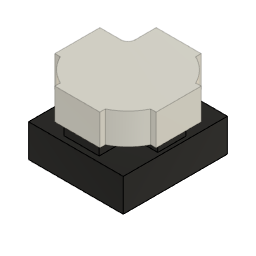
Marquardt_6425_0101 (Autodesk Fusion 360 design; units mm, degrees)
Autodesk Fusion 360 part; units mm, degrees
sketch "Sketch1" plane through (0, 0, 0) normal (0, 0, 1) x (1, 0, 0) in component "Base"
  line L0 (6.725, -7.4) -> (-6.725, -7.4)
  line L1 (-6.725, -7.4) -> (-6.725, 7.4)
  line L2 (-6.725, 7.4) -> (6.725, 7.4)
  line L3 (6.725, 7.4) -> (6.725, -7.4)
  line L4 (6.725, -7.4) -> (-6.725, 7.4) construction
  line L5 (-6.725, -7.4) -> (6.725, 7.4) construction
  dimension "d1" = 13.45
  dimension "d2" = 14.8
  constraint horizontal L0
  constraint perpendicular L0 L1
  constraint parallel L0 L2
  constraint parallel L1 L3
  constraint coincident L4 origin
  constraint coincident L5 origin
  measures "d1" distance of L1.end L2.end
  measures "d2" distance of L0.end L1.end
extrude "Extrude1" add sketch "Sketch1" along normal blind 4.65 makes body 1 in component "Base"
sketch "Sketch2" plane through (0, 0, 4.65) normal (0, 0, 1) x (-1, 0, 0) in component "Base"
  line L0 (-6.725, -7.4) -> (6.725, -7.4)
  line L1 (6.725, -7.4) -> (6.725, 7.4)
  line L2 (6.725, 7.4) -> (-6.725, 7.4)
  line L3 (-6.725, 7.4) -> (-6.725, -7.4)
  line L4 (0, -7.4) -> (0, 7.4) construction
  line L5 (6.725, 0) -> (-6.725, 0) construction
  line L6 (2.5, -6.6) -> (1.8392, -6.6)
  line L7 (1.8392, -6.6) -> (-2.5, -6.6)
  line L8 (-2.5, -6.6) -> (-2.5, -2)
  line L9 (-2.5, -2) -> (-6.225, -2)
  line L10 (-6.225, -2) -> (-6.225, 2)
  line L11 (-6.225, 2) -> (-2.5, 2)
  line L12 (-2.5, 2) -> (-2.5, 6.6)
  line L13 (-2.5, 6.6) -> (2.5, 6.6)
  line L14 (2.5, 6.6) -> (2.5, 2)
  line L15 (2.5, 2) -> (6.225, 2)
  line L16 (6.225, 2) -> (6.225, -2)
  line L17 (6.225, -2) -> (2.5, -2)
  line L18 (2.5, -2) -> (2.5, -6.6)
  dimension "d5" = 4
  dimension "d6" = 5
  dimension "d7" = 0.8
  dimension "d8" = 0.8
  dimension "d9" = 0.5
  constraint midpoint L0 L4.start
  constraint midpoint L2 L4.end
  constraint midpoint L1 L5.start
  constraint midpoint L3 L5.end
  constraint horizontal L6
  constraint perpendicular L4 L7
  constraint perpendicular L7 L8
  constraint perpendicular L8 L9
  constraint perpendicular L7 L10
  constraint perpendicular L10 L11
  constraint perpendicular L11 L12
  constraint perpendicular L10 L13
  constraint perpendicular L11 L14
  constraint perpendicular L14 L15
  constraint perpendicular L5 L16
  constraint perpendicular L16 L17
  constraint perpendicular L5 L18
  constraint equal L12 L14
  constraint equal L8 L18
  constraint equal L15 L17
  constraint equal L9 L15
  constraint equal L9 L11
  constraint symmetric L5 L9.end L10.end
  constraint symmetric L4 L12.end L13.end
  measures "d5" distance of L9.end L10.end
  measures "d6" distance of L12.end L13.end
  measures "d7" vertical distance of L2.end L12.end
  measures "d8" vertical distance of L0.start L7.end
  measures "d9" horizontal distance of L1.end L15.end
extrude "Extrude2" add sketch "Sketch2" along normal blind 4 contours L6 L7 L8 L9 L10 L11 L12 L13 L14 L15 L16 L17 L18 bodies 1 in component "Base"
sketch "Sketch3" plane through (0, 0, 0) normal (0, 0, -1) x (1, 0, 0) in component "Base"
  line L0 (-6.725, -7.4) -> (6.725, -7.4)
  line L1 (6.725, -7.4) -> (6.725, 7.4)
  line L2 (6.725, 7.4) -> (-6.725, 7.4)
  line L3 (-6.725, 7.4) -> (-6.725, -7.4)
  circle A0 centre (5.08, -5.08) radius 0.4
  circle A1 centre (-5.08, 5.08) radius 0.4
  dimension "d12" = 0.8
  dimension "d13" = 5.08
  dimension "d14" = 5.08
  dimension "d15" = 5.08
  dimension "d16" = 5.08
  constraint equal A0 A1
  measures "d12" diameter of A0
  measures "d13" horizontal distance of origin A0.centre
  measures "d14" vertical distance of origin A0.centre
  measures "d15" horizontal distance of origin A1.centre
  measures "d16" vertical distance of origin A1.centre
extrude "Extrude3" add sketch "Sketch3" along normal blind 1.5 contours A0 | A1 bodies 1 in component "Base"
chamfer "Chamfer1" distance 0.25 angle 45 2 edges at (-5.4529, -4.9354, -1.5) (4.7071, 5.2246, -1.5) on bodies 1 in component "Base"
sketch "Sketch4" plane through (0, 0, 4.65) normal (0, 0, 1) x (-1, 0, 0) in component "Base"
  line L0 (2.5, -2) -> (2.5, -6.6)
  line L1 (2.5, -6.6) -> (-2.5, -6.6)
  line L2 (-2.5, -6.6) -> (-2.5, -2)
  line L3 (-2.5, -2) -> (-6.225, -2)
  line L4 (-6.225, -2) -> (-6.225, 2)
  line L5 (-6.225, 2) -> (-2.5, 2)
  line L6 (-2.5, 2) -> (-2.5, 6.6)
  line L7 (-2.5, 6.6) -> (2.5, 6.6)
  line L8 (2.5, 6.6) -> (2.5, 2)
  line L9 (2.5, 2) -> (6.225, 2)
  line L10 (6.225, 2) -> (6.225, -2)
  line L11 (6.225, -2) -> (2.5, -2)
  line L12 (-6.725, -7.4) -> (6.725, -7.4)
  line L13 (6.725, -7.4) -> (6.725, 7.4)
  line L14 (6.725, 7.4) -> (-6.725, 7.4)
  line L15 (-6.725, 7.4) -> (-6.725, -7.4)
  circle A0 centre (4.15, -5.95) radius 0.5
  circle A1 centre (5.95, -4.15) radius 0.5
  dimension "d20" = 1
  dimension "d21" = 4.15
  dimension "d22" = 5.95
  dimension "d23" = 4.15
  dimension "d24" = 5.95
  constraint equal A0 A1
  measures "d20" diameter of A0
  measures "d21" horizontal distance of origin A0.centre
  measures "d22" horizontal distance of origin A1.centre
  measures "d23" vertical distance of origin A1.centre
  measures "d24" vertical distance of origin A0.centre
extrude "Extrude4" cut sketch "Sketch4" against normal through all contours A0 | A1 bodies 1 in component "Base"
ref_plane "WorkPlane1" through (0, 0, 10.7) normal (0, 0, -1) x (-1, 0, 0) in component "Plunger"
sketch "Sketch1 (2)" plane through (0, 0, 10.7) normal (0, 0, -1) x (1, 0, 0) in component "Plunger"
  line L0 (7.2, 7.2) -> (-7.2, 7.2) construction
  line L1 (-7.2, 7.2) -> (-7.2, -7.2) construction
  line L2 (-7.2, -7.2) -> (7.2, -7.2) construction
  line L3 (7.2, -7.2) -> (7.2, 7.2) construction
  line L4 (7.2, 7.2) -> (-7.2, -7.2) construction
  line L5 (-7.2, 7.2) -> (7.2, -7.2) construction
  line L6 (0, -7.2) -> (0, 7.2) construction
  line L7 (-7.2, 0) -> (7.2, 0) construction
  line L8 (-3.2, 7.2) -> (3.2, 7.2)
  line L9 (-3.2, -7.2) -> (3.2, -7.2)
  line L10 (7.2, -3.2) -> (7.2, 3.2)
  line L11 (-7.2, 3.2) -> (-7.2, -3.2)
  arc A0 (6.4219, 3.2) -> (3.2, 6.4219) centre (0, 0) ccw
  line L12 (7.2, 3.2) -> (6.4219, 3.2)
  line L13 (3.2, 7.2) -> (3.2, 6.4219)
  arc A1 (3.2, -6.4219) -> (6.4219, -3.2) centre (0, 0) ccw
  arc A2 (-3.2, 6.4219) -> (-6.4219, 3.2) centre (0, 0) ccw
  line L14 (-6.4219, 3.2) -> (-7.2, 3.2)
  line L15 (-3.2, 6.4219) -> (-3.2, 7.2)
  line L16 (6.4219, -3.2) -> (7.2, -3.2)
  line L17 (3.2, -6.4219) -> (3.2, -7.2)
  line L18 (-3.2, -7.2) -> (-3.2, -3.2)
  line L19 (-7.2, -3.2) -> (-3.2, -3.2)
  dimension "d33" = 14.4
  dimension "d34" = 14.4
  dimension "d35" = 6.4
  dimension "d36" = 6.4
  dimension "d37" = 6.4
  dimension "d38" = 6.4
  dimension "d39" = 7.175
  dimension "d40" = 0.7781
  dimension "d41" = 0.7781
  dimension "d42" = 7.175
  dimension "d43" = 7.175
  constraint horizontal L0
  constraint perpendicular L0 L1
  constraint parallel L0 L2
  constraint parallel L1 L3
  constraint coincident L4 A0.centre
  constraint coincident L5 A0.centre
  constraint coincident A0.centre A1.centre
  constraint midpoint L2 L6.start
  constraint midpoint L0 L6.end
  constraint midpoint L1 L7.start
  constraint midpoint L3 L7.end
  constraint horizontal L8
  constraint symmetric L6 L8.start L8.end
  constraint collinear L0 L8
  constraint coincident L2 L9.start
  constraint coincident L2 L9.end
  constraint parallel L2 L9
  constraint symmetric L6 L9.start L9.end
  constraint coincident L3 L10.start
  constraint coincident L3 L10.end
  constraint parallel L3 L10
  constraint coincident L1 L11.start
  constraint coincident L1 L11.end
  constraint perpendicular L7 L11
  constraint symmetric L7 L10.start L10.end
  constraint symmetric L7 L11.start L11.end
  constraint horizontal L12
  constraint vertical L13
  constraint vertical L17
  constraint horizontal L16
  constraint vertical L15
  constraint horizontal L14
  constraint perpendicular L9 L18
  constraint perpendicular L1 L19
  constraint coincident L18.end L19.end
  measures "d33" distance of L1.end L2.end
  measures "d34" distance of L0.end L1.end
  measures "d35" distance of L8.start L8.end
  measures "d36" distance of L9.start L9.end
  measures "d37" distance of L10.start L10.end
  measures "d38" distance of L11.start L11.end
  measures "d39" radius of A0
  measures "d40" distance of L8.end A0.end
  measures "d41" distance of L10.end A0.start
  measures "d42" radius of A1
  measures "d43" radius of A2
extrude "Extrude1'" add sketch "Sketch1 (2)" along normal blind 4.4 separate body makes body 2 in component "Plunger"
fillet "Fillet1" radius 1 1 edges at (-3.2, 3.2, 8.5) on bodies 2 in component "Plunger"
sketch "Sketch2 (2)" plane through (0, 0, 6.3) normal (0, 0, -1) x (1, 0, 0) in component "Plunger"
  arc A0 (-3.2, 6.4219) -> (-6.4219, 3.2) centre (0, 0) ccw
  line L0 (-6.4219, 3.2) -> (-7.2, 3.2)
  line L1 (-7.2, 3.2) -> (-7.2, -3.2)
  line L2 (-7.2, -3.2) -> (-4.2, -3.2)
  arc A1 (-3.2, -4.2) -> (-4.2, -3.2) centre (-4.2, -4.2) ccw
  line L3 (-3.2, -4.2) -> (-3.2, -7.2)
  line L4 (-3.2, -7.2) -> (3.2, -7.2)
  line L5 (3.2, -7.2) -> (3.2, -6.4219)
  arc A2 (3.2, -6.4219) -> (6.4219, -3.2) centre (0, 0) ccw
  line L6 (6.4219, -3.2) -> (7.2, -3.2)
  line L7 (7.2, -3.2) -> (7.2, 3.2)
  line L8 (7.2, 3.2) -> (6.4219, 3.2)
  arc A3 (6.4219, 3.2) -> (3.2, 6.4219) centre (0, 0) ccw
  line L9 (3.2, 6.4219) -> (3.2, 7.2)
  line L10 (3.2, 7.2) -> (-3.2, 7.2)
  line L11 (-3.2, 7.2) -> (-3.2, 6.4219)
  line L12 (-2.5, -2) -> (-6.225, -2)
  line L13 (-6.225, -2) -> (-6.225, 2)
  line L14 (-6.225, 2) -> (-2.5, 2)
  line L15 (-2.5, 2) -> (-2.5, 6.6)
  line L16 (-2.5, 6.6) -> (2.5, 6.6)
  line L17 (2.5, 6.6) -> (2.5, 2)
  line L18 (2.5, 2) -> (6.225, 2)
  line L19 (6.225, 2) -> (6.225, -2)
  line L20 (6.225, -2) -> (2.5, -2)
  line L21 (2.5, -2) -> (2.5, -6.6)
  line L22 (2.5, -6.6) -> (-2.5, -6.6)
  line L23 (-2.5, -6.6) -> (-2.5, -2)
extrude "Extrude2'" cut sketch "Sketch2 (2)" against normal blind 3.8 contours L12 L13 L14 L15 L16 L17 L18 L19 L20 L21 L22 L23 bodies 2 in component "Plunger"
sketch "Sketch1 (3)" plane through (0, 0, 0) normal (0, 0, -1) x (1, 0, 0) in component "PIns"
  circle A0 centre (-4.15, -5.95) radius 0.5
  circle A1 centre (-5.95, -4.15) radius 0.5
  circle A2 centre (-5.08, 5.08) radius 0.4
  circle A3 centre (5.08, -5.08) radius 0.4
  line L0 (-6.725, -7.4) -> (6.725, -7.4)
  line L1 (6.725, -7.4) -> (6.725, 7.4)
  line L2 (6.725, 7.4) -> (-6.725, 7.4)
  line L3 (-6.725, 7.4) -> (-6.725, -7.4)
  line L4 (0, 0) -> (0, -7.4) construction
  line L5 (0.45, -0.25) -> (-0.45, -0.25)
  line L6 (-0.45, -0.25) -> (-0.45, 0.25)
  line L7 (-0.45, 0.25) -> (0.45, 0.25)
  line L8 (0.45, 0.25) -> (0.45, -0.25)
  line L9 (0.45, -0.25) -> (-0.45, 0.25) construction
  line L10 (-0.45, -0.25) -> (0.45, 0.25) construction
  line L11 (0.45, -5.33) -> (-0.45, -5.33)
  line L12 (-0.45, -5.33) -> (-0.45, -4.83)
  line L13 (-0.45, -4.83) -> (0.45, -4.83)
  line L14 (0.45, -4.83) -> (0.45, -5.33)
  line L15 (0.45, -5.33) -> (-0.45, -4.83) construction
  line L16 (-0.45, -5.33) -> (0.45, -4.83) construction
  point P0 (0, -5.08)
  dimension "d50" = 0.9
  dimension "d51" = 0.5
  dimension "d52" = 0.5
  dimension "d53" = 0.9
  dimension "d54" = 5.08
  constraint coincident L4.start origin
  constraint midpoint L0 L4.end
  constraint horizontal L5
  constraint perpendicular L5 L6
  constraint parallel L5 L7
  constraint parallel L6 L8
  constraint coincident L9 L4.start
  constraint coincident L10 L4.start
  constraint horizontal L11
  constraint perpendicular L11 L12
  constraint parallel L11 L13
  constraint parallel L12 L14
  constraint coincident L15 P0
  constraint coincident L16 P0
  constraint coincident L4 P0
  measures "d50" distance of L6.end L7.end
  measures "d51" distance of L5.end L6.end
  measures "d52" distance of L11.end L12.end
  measures "d53" distance of L12.end L13.end
  measures "d54" distance of L4.start P0
extrude "Extrude1''" add sketch "Sketch1 (3)" along normal blind 3.6 separate body contours L5 L6 L7 L8 | L11 L12 L13 L14 makes body 3 at (0.15, 0.25, -1.2) makes body 4 at (-0.15, 4.83, -1.2) in component "PIns"
chamfer "Chamfer1'" distance 0.3 angle 45 4 edges at (-0.45, 0, -3.6) (0.45, 0, -3.6) (-0.45, 5.08, -3.6) (0.45, 5.08, -3.6) on bodies 3 4 in component "PIns"
component "Base" placed x (1, 0, 0) y (0, 1, 0) z (0, 0, 1) at (0, 0, 0)
component "Plunger" placed x (1, 0, 0) y (0, 1, 0) z (0, 0, 1) at (0, 0, 0)
component "PIns" placed x (1, 0, 0) y (0, 1, 0) z (0, 0, 1) at (0, 0, 0)
equation "d8 = d7"
equation "d15 = d13"
equation "d16 = d14"
equation "d36 = d35"
equation "d37 = d35"
equation "d38 = d35"
equation "d42 = d39"
equation "d43 = d39"
equation "d52 = d51"
equation "d53 = d50"
